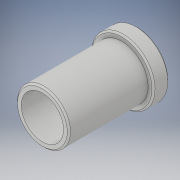
# Autodesk Inventor part: Component 5(Ram Bearing)
Saved by Autodesk Inventor 2018 (Build 220112000, 112)
## iProperties
Created: 2023-03-14
Part Number: Component 5(Ram Bearing)
Material: Generic
Document SubType Name: Modeling
Designer: Habib Mohamed
Density: 1 g/cm^3
Appearance: Default
Author: Habib Mohamed
Autodesk Inventor part; units mm, degrees
ref_plane "YZ Plane" through (0, 0, 0) normal (1, 0, 0) x (0, 1, 0)
ref_plane "XZ Plane" through (0, 0, 0) normal (0, 1, 0) x (-1, 0, 0)
ref_plane "XY Plane" through (0, 0, 0) normal (0, 0, 1) x (1, 0, 0)
sketch "Sketch1" plane through (0, 0, 0) normal (1, 0, 0) x (0, 1, 0)
  line L0 (0, 0) -> (0, -9) construction
  line L1 (2, 0) -> (2, -9)
  line L2 (2, -9) -> (3, -9)
  line L3 (3, -9) -> (3, -7.5)
  line L4 (3, -7.5) -> (2.5, -7.5)
  line L5 (2.5, -7.5) -> (2.5, 0)
  line L6 (2.5, 0) -> (2, 0)
  line L7 (0, 0) -> (7.91, 0) construction
  dimension "d0" = 9
  dimension "d1" = 2
  dimension "d2" = 2.5
  dimension "d3" = 3
  dimension "d4" = 1.5
  dimension "d5" = 9
  constraints: 16 end point, 4 perpendicular, 2 horizontal, 2 vertical, 1 collinear
  measures "d0" distance of L0.start L0.end
  measures "d1" distance between parallel lines of L0 L1
  measures "d2" distance between parallel lines of L0 L5
  measures "d3" distance between parallel lines of L0 L3
  measures "d4" distance of L2.end L3.end
  measures "d5" distance between parallel lines of L2 L6
revolve "Revolution1" add sketch "Sketch1" angle 360 about axis through (0, 0, 0) along (0, 0, -1)
chamfer "Chamfer1" distance 0.15 angle 45 3 edges at (0, -3, -7.5) (0, -3, -9) (0, -2.5, 0)
body "Solid1"
